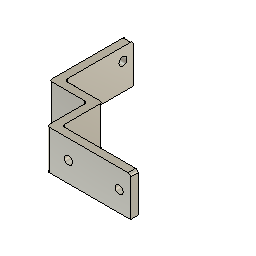
Right-Angled_Daughterboard_Bracket_v1 (Autodesk Fusion 360 design; units mm, degrees)
Autodesk Fusion 360 part; units mm, degrees
sketch "Sketch1" plane through (0, 0, 0) normal (1, 0, 0) x (0, 1, 0)
  line L0 (0, 0) -> (-30, 0)
  line L1 (-30, 0) -> (-30, 15.5)
  line L2 (-30, 15.5) -> (0, 15.5)
  line L3 (0, 15.5) -> (0, 0)
  circle A0 centre (-4, 10.5) radius 1.6
  circle A1 centre (-24, 10.5) radius 1.6
  dimension "d1" = 30
  dimension "d2" = 15.5
  dimension "d3" = 3.2
  dimension "d4" = 3.2
  dimension "d5" = 20
  dimension "d6" = 4
  dimension "d7" = 5
  constraint horizontal L0
  constraint vertical L1
  constraint horizontal L2
  constraint vertical L3
  constraint coincident L0.start L3.end
  measures "d1" distance of L0.start L0.end
  measures "d2" distance of L0.start L2.end
  measures "d3" diameter of A0
  measures "d4" diameter of A1
  measures "d5" distance of A0.centre A1.centre
  measures "d6" distance of L3 A0.centre
  measures "d7" distance of L2 A0.centre
extrude "Extrude1" add sketch "Sketch1" along normal blind 3 makes body 1
sketch "Sketch2" plane through (0, 0, 0) normal (0, 1, 0) x (1, 0, 0)
sketch "Sketch3" plane through (0, -30, 0) normal (0, -1, 0) x (1, 0, 0)
  line L0 (0, 15.5) -> (0, 0)
  line L1 (0, 0) -> (3, 0)
  line L2 (3, 0) -> (3, 15.5)
  line L3 (3, 15.5) -> (0, 15.5)
  line L4 (3, 15.5) -> (15, 15.5)
  line L5 (15, 15.5) -> (15, 0)
  line L6 (15, 0) -> (3, 0)
  line L7 (3, 0) -> (3, 15.5)
  dimension "d10" = 12
  constraint horizontal L4
  constraint vertical L5
  constraint horizontal L6
  constraint vertical L7
  constraint coincident L2.end L3.start
  measures "d10" distance of L2.end L4.end
extrude "Extrude2" add sketch "Sketch3" against normal blind 3 contours L2 L4 L5 L6 L7 bodies 1
sketch "Sketch4" plane through (15, 0, 0) normal (1, 0, 0) x (0, 1, 0)
  line L0 (-30, 15.5) -> (-30, 0)
  line L1 (-30, 0) -> (-27, 0)
  line L2 (-27, 0) -> (-27, 15.5)
  line L3 (-27, 15.5) -> (-30, 15.5)
  line L4 (-30, 15.5) -> (-43, 15.5)
  line L5 (-43, 15.5) -> (-43, 0)
  line L6 (-43, 0) -> (-30, 0)
  line L7 (-30, 0) -> (-30, 15.5)
  dimension "d13" = 13
  constraint horizontal L4
  constraint vertical L5
  constraint horizontal L6
  constraint vertical L7
  constraint coincident L0.start L3.end
  measures "d13" distance of L0.start L4.end
extrude "Extrude3" add sketch "Sketch4" along normal blind 3 separate body contours L0 L4 L5 L6 L7 makes body 2
extrude "Extrude4" add 1 faces at (16, -30, 10.3333) along direction (0, 1, 0) blind 3 on bodies 2 bodies 2 1
fillet "Fillet1" radius 1 1 edges at (18, -27, 7.75) on bodies 2
fillet "Fillet2" radius 1 1 edges at (3, -27, 7.75) on bodies 2
fillet "Fillet3" radius 1 1 edges at (1.5, 0, 15.5) on bodies 2
fillet "Fillet4" radius 1 1 edges at (0, -30, 7.75) on bodies 2
fillet "Fillet5" radius 1 1 edges at (15, -30, 7.75) on bodies 2
sketch "Sketch13" plane through (0, -43, 0) normal (0, -1, 0) x (1, 0, 0)
  line L0 (15, 15.5) -> (15, 0)
  line L1 (15, 0) -> (18, 0)
  line L2 (18, 0) -> (18, 15.5)
  line L3 (18, 15.5) -> (15, 15.5)
  line L4 (15, 15.5) -> (46, 15.5)
  line L5 (46, 15.5) -> (46, 0)
  line L6 (46, 0) -> (15, 0)
  line L7 (15, 0) -> (15, 15.5)
  circle A0 centre (43.5, 8) radius 1.6
  circle A1 centre (23.5, 8) radius 1.6
  line L8 (15, 15.5) -> (15, 0)
  line L9 (15, 0) -> (18, 0)
  line L10 (18, 0) -> (18, 15.5)
  line L11 (18, 15.5) -> (15, 15.5)
  dimension "d97" = 31
  dimension "d98" = 15.5
  dimension "d99" = 3.2
  dimension "d101" = 3.2
  dimension "d102" = 20
  dimension "d111" = 7.5
  dimension "d114" = 2.5
  constraint horizontal L4
  constraint vertical L5
  constraint horizontal L6
  constraint vertical L7
  constraint coincident L0.start L3.end
  measures "d97" distance of L0.start L4.end
  measures "d98" distance of L0.start L0.end
  measures "d99" diameter of A0
  measures "d101" diameter of A1
  measures "d102" distance of A0.centre A1.centre
  measures "d111" distance of L4 A0.centre
  measures "d114" distance of L5 A0.centre
extrude "Extrude19" add sketch "Sketch13" along normal blind 3 contours L2 L4 L5 L6 L10 bodies 2
extrude "Extrude20" add 1 faces at (18, -44, 5.1667) along direction (-1, 0, 0) blind 3 on bodies 2 bodies 2
fillet "Fillet8" radius 1 1 edges at (15, -46, 7.75) on bodies 2
fillet "Fillet9" radius 1 1 edges at (18, -43, 7.75) on bodies 2
extrude "Extrude21" add 1 faces at (46, -44, 10.3333) along direction (1, 0, 0) blind 2 on bodies 2 bodies 2
fillet "Fillet11" radius 1 1 edges at (48, -44.5, 15.5) on bodies 2
